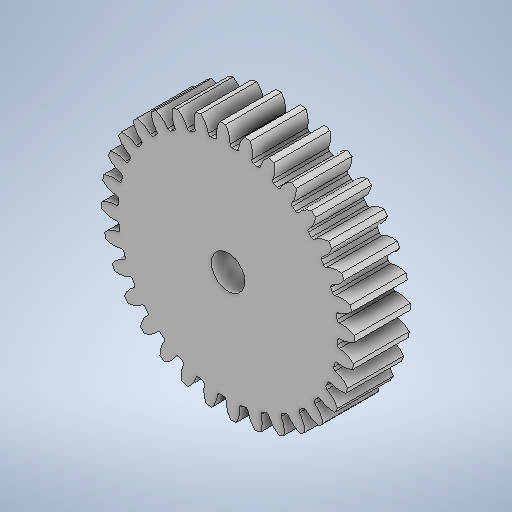
# Autodesk Inventor part: gear32
Saved by Autodesk Inventor 2025.1 (Build 291241000, 241)
## iProperties
Created: 2024-11-04
Part Number: gear32
Material: Generic
Document SubType Name: Modeling
Designer: rishi
Density: 1 g/cm^3
Appearance: Default
Author: rishi
Autodesk Inventor part; units mm, degrees
ref_plane "YZ Plane" through (0, 0, 0) normal (1, 0, 0) x (0, 1, 0)
ref_plane "XZ Plane" through (0, 0, 0) normal (0, 1, 0) x (-1, 0, 0)
ref_plane "XY Plane" through (0, 0, 0) normal (0, 0, 1) x (1, 0, 0)
sketch "Sketch1" plane through (0, 0, 0) normal (0, 0, 1) x (1, 0, 0)
  arc A0 (0.375172, 28.714431) -> (0.375938, 28.717754) centre (-5.995256, 30.18306) ccw
  arc A1 (0.541208, 30.065293) -> (-0.682771, 33.993144) centre (-5.995256, 30.18306) ccw
  arc A2 (0.541208, 30.065293) -> (1.115535, 29.478901) centre (1.111711, 30.049607) ccw
  arc A3 (0.255749, 26.188813) -> (0.375172, 26.259051) centre (-2.99886, 31.859172) ccw
  arc A4 (-2.20376, 33.928505) -> (-3.090042, 29.910974) centre (3.413346, 30.582826) ccw
  arc A5 (-3.587273, 29.281077) -> (-3.090042, 29.910974) centre (-3.656607, 29.84701) ccw
  arc A6 (-3.031796, 29.343794) -> (-3.031451, 29.343829) centre (-3.090042, 29.910974) ccw
  arc A7 (-0.682771, 33.993144) -> (-2.20376, 33.928505) centre (0, 0) ccw
  arc A8 (-0.682771, 33.993144) -> (-2.20376, 33.928505) centre (0, 0) ccw
  arc A9 (-11.19341, 27.293911) -> (-11.334874, 27.235466) centre (0, 0) ccw
  arc A10 (1.115535, 29.478901) -> (-3.587273, 29.281077) centre (0, 0) ccw
  arc A11 (-7.301386, 33.206773) -> (-8.780538, 32.846646) centre (0, 0) ccw
  arc A12 (-5.334639, 29.593181) -> (-7.301386, 33.206773) centre (-11.768482, 28.433485) ccw
  arc A13 (-5.334639, 29.593181) -> (-4.656948, 29.130102) centre (-4.772037, 29.689096) ccw
  arc A14 (-4.656948, 29.130102) -> (-9.2308, 28.018607) centre (0, 0) ccw
  arc A15 (-9.2308, 28.018607) -> (-8.866009, 28.733406) centre (-9.409209, 28.560139) ccw
  arc A16 (-8.780538, 32.846646) -> (-8.866009, 28.733406) centre (-2.618654, 30.661097) ccw
  arc A17 (-13.639412, 31.144284) -> (-15.019885, 30.502509) centre (0, 0) ccw
  arc A18 (-11.005479, 27.98382) -> (-13.639412, 31.144284) centre (-17.089451, 25.591226) ccw
  arc A19 (-11.005479, 27.98382) -> (-10.250467, 27.66185) centre (-10.472399, 28.18765) ccw
  arc A20 (-10.250467, 27.66185) -> (-14.519591, 25.679398) centre (0, 0) ccw
  arc A21 (-14.519591, 25.679398) -> (-14.301261, 26.451629) centre (-14.80022, 26.175719) ccw
  arc A22 (-15.019885, 30.502509) -> (-14.301261, 26.451629) centre (-8.55002, 29.561078) ccw
  arc A23 (-19.453283, 27.884939) -> (-20.682027, 26.986177) centre (0, 0) ccw
  arc A24 (-16.253384, 25.299057) -> (-19.453283, 27.884939) centre (-21.753683, 21.765511) ccw
  arc A25 (-16.253384, 25.299057) -> (-15.450066, 25.130568) centre (-15.770313, 25.602968) ccw
  arc A26 (-15.450066, 25.130568) -> (-19.250403, 22.353344) centre (0, 0) ccw
  arc A27 (-19.250403, 22.353344) -> (-19.186923, 23.153331) centre (-19.622467, 22.78538) ccw
  arc A28 (-20.682027, 26.986177) -> (-19.186923, 23.153331) centre (-14.152814, 27.325044) ccw
  arc A29 (-24.519575, 23.55399) -> (-25.549369, 22.432782) centre (0, 0) ccw
  arc A30 (-20.876681, 21.642065) -> (-24.519575, 23.55399) centre (-25.581932, 17.10336) ccw
  arc A31 (-20.876681, 21.642065) -> (-20.055928, 21.633533) centre (-20.462182, 22.034379) ccw
  arc A32 (-20.055928, 21.633533) -> (-23.241433, 18.168263) centre (0, 0) ccw
  arc A33 (-23.241433, 18.168263) -> (-23.335243, 18.965263) centre (-23.690634, 18.519412) ccw
  arc A34 (-25.549369, 22.432782) -> (-23.335243, 18.965263) centre (-19.211724, 24.038924) ccw
  arc A35 (-28.643594, 18.317875) -> (-29.434864, 17.017308) centre (0, 0) ccw
  arc A36 (-24.697699, 17.15338) -> (-28.643594, 18.317875) centre (-28.427083, 11.783937) ccw
  arc A37 (-24.697699, 17.15338) -> (-23.891052, 17.305133) centre (-24.367701, 17.619021) ccw
  arc A38 (-23.891052, 17.305133) -> (-26.339308, 13.284986) centre (0, 0) ccw
  arc A39 (-26.339308, 13.284986) -> (-26.586802, 14.048371) centre (-26.848383, 13.541753) ccw
  arc A40 (-29.434864, 17.017308) -> (-26.586802, 14.048371) centre (-23.532337, 19.829002) ccw
  arc A41 (-31.666855, 12.377814) -> (-32.189194, 10.947868) centre (0, 0) ccw
  arc A42 (-27.569598, 12.005501) -> (-31.666855, 12.377814) centre (-30.179796, 6.011663) ccw
  arc A43 (-27.569598, 12.005501) -> (-26.808056, 12.311707) centre (-27.336783, 12.526574) ccw
  arc A44 (-26.808056, 12.311707) -> (-28.424978, 7.891175) centre (0, 0) ccw
  arc A45 (-28.424978, 7.891175) -> (-28.816645, 8.591608) centre (-28.974364, 8.043692) ccw
  arc A46 (-32.189194, 10.947868) -> (-28.816645, 8.591608) centre (-26.948616, 14.857062) ccw
  arc A47 (-33.473177, 5.962081) -> (-33.70651, 4.457708) centre (0, 0) ccw
  arc A48 (-29.382012, 6.396257) -> (-33.473177, 5.962081) centre (-30.772717, 0.008364) ccw
  arc A49 (-29.382012, 6.396257) -> (-28.694842, 6.845149) centre (-29.255328, 6.952737) ccw
  arc A50 (-28.694842, 6.845149) -> (-29.418292, 2.19411) centre (0, 0) ccw
  arc A51 (-29.418292, 2.19411) -> (-29.939081, 2.804674) centre (-29.986876, 2.236517) ccw
  arc A52 (-33.70651, 4.457708) -> (-29.939081, 2.804674) centre (-29.329275, 9.314173) ccw
  arc A53 (-33.993144, -0.682771) -> (-33.928505, -2.20376) centre (0, 0) ccw
  arc A54 (-30.065293, 0.541208) -> (-33.993144, -0.682771) centre (-30.18306, -5.995256) ccw
  arc A55 (-30.065293, 0.541208) -> (-29.478901, 1.115535) centre (-30.049607, 1.111711) ccw
  arc A56 (-29.478901, 1.115535) -> (-29.281077, -3.587273) centre (0, 0) ccw
  arc A57 (-29.281077, -3.587273) -> (-29.910974, -3.090042) centre (-29.84701, -3.656607) ccw
  arc A58 (-33.928505, -2.20376) -> (-29.910974, -3.090042) centre (-30.582826, 3.413346) ccw
  arc A59 (-33.206773, -7.301386) -> (-32.846646, -8.780538) centre (0, 0) ccw
  arc A60 (-29.593181, -5.334639) -> (-33.206773, -7.301386) centre (-28.433485, -11.768482) ccw
  arc A61 (-29.593181, -5.334639) -> (-29.130102, -4.656948) centre (-29.689096, -4.772037) ccw
  arc A62 (-29.130102, -4.656948) -> (-28.018607, -9.2308) centre (0, 0) ccw
  arc A63 (-28.018607, -9.2308) -> (-28.733406, -8.866009) centre (-28.560139, -9.409209) ccw
  arc A64 (-32.846646, -8.780538) -> (-28.733406, -8.866009) centre (-30.661097, -2.618654) ccw
  arc A65 (-31.144284, -13.639412) -> (-30.502509, -15.019885) centre (0, 0) ccw
  arc A66 (-27.98382, -11.005479) -> (-31.144284, -13.639412) centre (-25.591226, -17.089451) ccw
  arc A67 (-27.98382, -11.005479) -> (-27.66185, -10.250467) centre (-28.18765, -10.472399) ccw
  arc A68 (-27.66185, -10.250467) -> (-25.679398, -14.519591) centre (0, 0) ccw
  arc A69 (-25.679398, -14.519591) -> (-26.451629, -14.301261) centre (-26.175719, -14.80022) ccw
  arc A70 (-30.502509, -15.019885) -> (-26.451629, -14.301261) centre (-29.561078, -8.55002) ccw
  arc A71 (-27.884939, -19.453283) -> (-26.986177, -20.682027) centre (0, 0) ccw
  arc A72 (-25.299057, -16.253384) -> (-27.884939, -19.453283) centre (-21.765511, -21.753683) ccw
  arc A73 (-25.299057, -16.253384) -> (-25.130568, -15.450066) centre (-25.602968, -15.770313) ccw
  arc A74 (-25.130568, -15.450066) -> (-22.353344, -19.250403) centre (0, 0) ccw
  arc A75 (-22.353344, -19.250403) -> (-23.153331, -19.186923) centre (-22.78538, -19.622467) ccw
  arc A76 (-26.986177, -20.682027) -> (-23.153331, -19.186923) centre (-27.325044, -14.152814) ccw
  arc A77 (-23.55399, -24.519575) -> (-22.432782, -25.549369) centre (0, 0) ccw
  arc A78 (-21.642065, -20.876681) -> (-23.55399, -24.519575) centre (-17.10336, -25.581932) ccw
  arc A79 (-21.642065, -20.876681) -> (-21.633533, -20.055928) centre (-22.034379, -20.462182) ccw
  arc A80 (-21.633533, -20.055928) -> (-18.168263, -23.241433) centre (0, 0) ccw
  arc A81 (-18.168263, -23.241433) -> (-18.965263, -23.335243) centre (-18.519412, -23.690634) ccw
  arc A82 (-22.432782, -25.549369) -> (-18.965263, -23.335243) centre (-24.038924, -19.211724) ccw
  arc A83 (-18.317875, -28.643594) -> (-17.017308, -29.434864) centre (0, 0) ccw
  arc A84 (-17.15338, -24.697699) -> (-18.317875, -28.643594) centre (-11.783937, -28.427083) ccw
  arc A85 (-17.15338, -24.697699) -> (-17.305133, -23.891052) centre (-17.619021, -24.367701) ccw
  arc A86 (-17.305133, -23.891052) -> (-13.284986, -26.339308) centre (0, 0) ccw
  arc A87 (-13.284986, -26.339308) -> (-14.048371, -26.586802) centre (-13.541753, -26.848383) ccw
  arc A88 (-17.017308, -29.434864) -> (-14.048371, -26.586802) centre (-19.829002, -23.532337) ccw
  arc A89 (-12.377814, -31.666855) -> (-10.947868, -32.189194) centre (0, 0) ccw
  arc A90 (-12.005501, -27.569598) -> (-12.377814, -31.666855) centre (-6.011663, -30.179796) ccw
  arc A91 (-12.005501, -27.569598) -> (-12.311707, -26.808056) centre (-12.526574, -27.336783) ccw
  arc A92 (-12.311707, -26.808056) -> (-7.891175, -28.424978) centre (0, 0) ccw
  arc A93 (-7.891175, -28.424978) -> (-8.591608, -28.816645) centre (-8.043692, -28.974364) ccw
  arc A94 (-10.947868, -32.189194) -> (-8.591608, -28.816645) centre (-14.857062, -26.948616) ccw
  arc A95 (-5.962081, -33.473177) -> (-4.457708, -33.70651) centre (0, 0) ccw
  arc A96 (-6.396257, -29.382012) -> (-5.962081, -33.473177) centre (-0.008364, -30.772717) ccw
  arc A97 (-6.396257, -29.382012) -> (-6.845149, -28.694842) centre (-6.952737, -29.255328) ccw
  arc A98 (-6.845149, -28.694842) -> (-2.19411, -29.418292) centre (0, 0) ccw
  arc A99 (-2.19411, -29.418292) -> (-2.804674, -29.939081) centre (-2.236517, -29.986876) ccw
  arc A100 (-4.457708, -33.70651) -> (-2.804674, -29.939081) centre (-9.314173, -29.329275) ccw
  arc A101 (0.682771, -33.993144) -> (2.20376, -33.928505) centre (0, 0) ccw
  arc A102 (-0.541208, -30.065293) -> (0.682771, -33.993144) centre (5.995256, -30.18306) ccw
  arc A103 (-0.541208, -30.065293) -> (-1.115535, -29.478901) centre (-1.111711, -30.049607) ccw
  arc A104 (-1.115535, -29.478901) -> (3.587273, -29.281077) centre (0, 0) ccw
  arc A105 (3.587273, -29.281077) -> (3.090042, -29.910974) centre (3.656607, -29.84701) ccw
  arc A106 (2.20376, -33.928505) -> (3.090042, -29.910974) centre (-3.413346, -30.582826) ccw
  arc A107 (7.301386, -33.206773) -> (8.780538, -32.846646) centre (0, 0) ccw
  arc A108 (5.334639, -29.593181) -> (7.301386, -33.206773) centre (11.768482, -28.433485) ccw
  arc A109 (5.334639, -29.593181) -> (4.656948, -29.130102) centre (4.772037, -29.689096) ccw
  arc A110 (4.656948, -29.130102) -> (9.2308, -28.018607) centre (0, 0) ccw
  arc A111 (9.2308, -28.018607) -> (8.866009, -28.733406) centre (9.409209, -28.560139) ccw
  arc A112 (8.780538, -32.846646) -> (8.866009, -28.733406) centre (2.618654, -30.661097) ccw
  arc A113 (13.639412, -31.144284) -> (15.019885, -30.502509) centre (0, 0) ccw
  arc A114 (11.005479, -27.98382) -> (13.639412, -31.144284) centre (17.089451, -25.591226) ccw
  arc A115 (11.005479, -27.98382) -> (10.250467, -27.66185) centre (10.472399, -28.18765) ccw
  arc A116 (10.250467, -27.66185) -> (14.519591, -25.679398) centre (0, 0) ccw
  arc A117 (14.519591, -25.679398) -> (14.301261, -26.451629) centre (14.80022, -26.175719) ccw
  arc A118 (15.019885, -30.502509) -> (14.301261, -26.451629) centre (8.55002, -29.561078) ccw
  arc A119 (19.453283, -27.884939) -> (20.682027, -26.986177) centre (0, 0) ccw
  arc A120 (16.253384, -25.299057) -> (19.453283, -27.884939) centre (21.753683, -21.765511) ccw
  arc A121 (16.253384, -25.299057) -> (15.450066, -25.130568) centre (15.770313, -25.602968) ccw
  arc A122 (15.450066, -25.130568) -> (19.250403, -22.353344) centre (0, 0) ccw
  arc A123 (19.250403, -22.353344) -> (19.186923, -23.153331) centre (19.622467, -22.78538) ccw
  arc A124 (20.682027, -26.986177) -> (19.186923, -23.153331) centre (14.152814, -27.325044) ccw
  arc A125 (24.519575, -23.55399) -> (25.549369, -22.432782) centre (0, 0) ccw
  arc A126 (20.876681, -21.642065) -> (24.519575, -23.55399) centre (25.581932, -17.10336) ccw
  arc A127 (20.876681, -21.642065) -> (20.055928, -21.633533) centre (20.462182, -22.034379) ccw
  arc A128 (20.055928, -21.633533) -> (23.241433, -18.168263) centre (0, 0) ccw
  arc A129 (23.241433, -18.168263) -> (23.335243, -18.965263) centre (23.690634, -18.519412) ccw
  arc A130 (25.549369, -22.432782) -> (23.335243, -18.965263) centre (19.211724, -24.038924) ccw
  arc A131 (28.643594, -18.317875) -> (29.434864, -17.017308) centre (0, 0) ccw
  arc A132 (24.697699, -17.15338) -> (28.643594, -18.317875) centre (28.427083, -11.783937) ccw
  arc A133 (24.697699, -17.15338) -> (23.891052, -17.305133) centre (24.367701, -17.619021) ccw
  arc A134 (23.891052, -17.305133) -> (26.339308, -13.284986) centre (0, 0) ccw
  arc A135 (26.339308, -13.284986) -> (26.586802, -14.048371) centre (26.848383, -13.541753) ccw
  arc A136 (29.434864, -17.017308) -> (26.586802, -14.048371) centre (23.532337, -19.829002) ccw
  arc A137 (31.666855, -12.377814) -> (32.189194, -10.947868) centre (0, 0) ccw
  arc A138 (27.569598, -12.005501) -> (31.666855, -12.377814) centre (30.179796, -6.011663) ccw
  arc A139 (27.569598, -12.005501) -> (26.808056, -12.311707) centre (27.336783, -12.526574) ccw
  arc A140 (26.808056, -12.311707) -> (28.424978, -7.891175) centre (0, 0) ccw
  arc A141 (28.424978, -7.891175) -> (28.816645, -8.591608) centre (28.974364, -8.043692) ccw
  arc A142 (32.189194, -10.947868) -> (28.816645, -8.591608) centre (26.948616, -14.857062) ccw
  arc A143 (33.473177, -5.962081) -> (33.70651, -4.457708) centre (0, 0) ccw
  arc A144 (29.382012, -6.396257) -> (33.473177, -5.962081) centre (30.772717, -0.008364) ccw
  arc A145 (29.382012, -6.396257) -> (28.694842, -6.845149) centre (29.255328, -6.952737) ccw
  arc A146 (28.694842, -6.845149) -> (29.418292, -2.19411) centre (0, 0) ccw
  arc A147 (29.418292, -2.19411) -> (29.939081, -2.804674) centre (29.986876, -2.236517) ccw
  arc A148 (33.70651, -4.457708) -> (29.939081, -2.804674) centre (29.329275, -9.314173) ccw
  arc A149 (33.993144, 0.682771) -> (33.928505, 2.20376) centre (0, 0) ccw
  arc A150 (30.065293, -0.541208) -> (33.993144, 0.682771) centre (30.18306, 5.995256) ccw
  arc A151 (30.065293, -0.541208) -> (29.478901, -1.115535) centre (30.049607, -1.111711) ccw
  arc A152 (29.478901, -1.115535) -> (29.281077, 3.587273) centre (0, 0) ccw
  arc A153 (29.281077, 3.587273) -> (29.910974, 3.090042) centre (29.84701, 3.656607) ccw
  arc A154 (33.928505, 2.20376) -> (29.910974, 3.090042) centre (30.582826, -3.413346) ccw
  arc A155 (33.206773, 7.301386) -> (32.846646, 8.780538) centre (0, 0) ccw
  arc A156 (29.593181, 5.334639) -> (33.206773, 7.301386) centre (28.433485, 11.768482) ccw
  arc A157 (29.593181, 5.334639) -> (29.130102, 4.656948) centre (29.689096, 4.772037) ccw
  arc A158 (29.130102, 4.656948) -> (28.018607, 9.2308) centre (0, 0) ccw
  arc A159 (28.018607, 9.2308) -> (28.733406, 8.866009) centre (28.560139, 9.409209) ccw
  arc A160 (32.846646, 8.780538) -> (28.733406, 8.866009) centre (30.661097, 2.618654) ccw
  arc A161 (31.144284, 13.639412) -> (30.502509, 15.019885) centre (0, 0) ccw
  arc A162 (27.98382, 11.005479) -> (31.144284, 13.639412) centre (25.591226, 17.089451) ccw
  arc A163 (27.98382, 11.005479) -> (27.66185, 10.250467) centre (28.18765, 10.472399) ccw
  arc A164 (27.66185, 10.250467) -> (25.679398, 14.519591) centre (0, 0) ccw
  arc A165 (25.679398, 14.519591) -> (26.451629, 14.301261) centre (26.175719, 14.80022) ccw
  arc A166 (30.502509, 15.019885) -> (26.451629, 14.301261) centre (29.561078, 8.55002) ccw
  arc A167 (27.884939, 19.453283) -> (26.986177, 20.682027) centre (0, 0) ccw
  arc A168 (25.299057, 16.253384) -> (27.884939, 19.453283) centre (21.765511, 21.753683) ccw
  arc A169 (25.299057, 16.253384) -> (25.130568, 15.450066) centre (25.602968, 15.770313) ccw
  arc A170 (25.130568, 15.450066) -> (22.353344, 19.250403) centre (0, 0) ccw
  arc A171 (22.353344, 19.250403) -> (23.153331, 19.186923) centre (22.78538, 19.622467) ccw
  arc A172 (26.986177, 20.682027) -> (23.153331, 19.186923) centre (27.325044, 14.152814) ccw
  arc A173 (23.55399, 24.519575) -> (22.432782, 25.549369) centre (0, 0) ccw
  arc A174 (21.642065, 20.876681) -> (23.55399, 24.519575) centre (17.10336, 25.581932) ccw
  arc A175 (21.642065, 20.876681) -> (21.633533, 20.055928) centre (22.034379, 20.462182) ccw
  arc A176 (21.633533, 20.055928) -> (18.168263, 23.241433) centre (0, 0) ccw
  arc A177 (18.168263, 23.241433) -> (18.965263, 23.335243) centre (18.519412, 23.690634) ccw
  arc A178 (22.432782, 25.549369) -> (18.965263, 23.335243) centre (24.038924, 19.211724) ccw
  arc A179 (18.317875, 28.643594) -> (17.017308, 29.434864) centre (0, 0) ccw
  arc A180 (17.15338, 24.697699) -> (18.317875, 28.643594) centre (11.783937, 28.427083) ccw
  arc A181 (17.15338, 24.697699) -> (17.305133, 23.891052) centre (17.619021, 24.367701) ccw
  arc A182 (17.305133, 23.891052) -> (13.284986, 26.339308) centre (0, 0) ccw
  arc A183 (13.284986, 26.339308) -> (14.048371, 26.586802) centre (13.541753, 26.848383) ccw
  arc A184 (17.017308, 29.434864) -> (14.048371, 26.586802) centre (19.829002, 23.532337) ccw
  arc A185 (12.377814, 31.666855) -> (10.947868, 32.189194) centre (0, 0) ccw
  arc A186 (12.005501, 27.569598) -> (12.377814, 31.666855) centre (6.011663, 30.179796) ccw
  arc A187 (12.005501, 27.569598) -> (12.311707, 26.808056) centre (12.526574, 27.336783) ccw
  arc A188 (12.311707, 26.808056) -> (7.891175, 28.424978) centre (0, 0) ccw
  arc A189 (7.891175, 28.424978) -> (8.591608, 28.816645) centre (8.043692, 28.974364) ccw
  arc A190 (10.947868, 32.189194) -> (8.591608, 28.816645) centre (14.857062, 26.948616) ccw
  arc A191 (5.962081, 33.473177) -> (4.457708, 33.70651) centre (0, 0) ccw
  arc A192 (6.396257, 29.382012) -> (5.962081, 33.473177) centre (0.008364, 30.772717) ccw
  arc A193 (6.396257, 29.382012) -> (6.845149, 28.694842) centre (6.952737, 29.255328) ccw
  arc A194 (6.845149, 28.694842) -> (2.19411, 29.418292) centre (0, 0) ccw
  arc A195 (2.19411, 29.418292) -> (2.804674, 29.939081) centre (2.236517, 29.986876) ccw
  arc A196 (4.457708, 33.70651) -> (2.804674, 29.939081) centre (9.314173, 29.329275) ccw
  circle A197 centre (0, 0) radius 29.5
  arc A198 (3.5, 2.828427) -> (3.5, -2.828427) centre (0, 0) ccw
  line L0 (3.5, -2.828427) -> (3.5, 2.828427)
  point P0 (0, 34)
  point P1 (0, 34)
  point P2 (0, 32.79)
  point P3 (-6.397012, 32.159949)
  point P4 (-8.6979, 28.188589)
  point P5 (-12.54819, 30.29401)
  point P6 (-14.030093, 25.950077)
  point P7 (-18.217148, 27.263889)
  point P8 (-18.823118, 22.714318)
  point P9 (-23.186031, 23.186031)
  point P10 (-22.89278, 18.605661)
  point P11 (-27.263889, 18.217148)
  point P12 (-26.082686, 13.781998)
  point P13 (-30.29401, 12.54819)
  point P14 (-28.270249, 8.428701)
  point P15 (-32.159949, 6.397012)
  point P16 (-29.371402, 2.751494)
  point P17 (-32.79, 0)
  point P18 (-29.343829, -3.031451)
  point P19 (-32.159949, -6.397012)
  point P20 (-28.188589, -8.6979)
  point P21 (-30.29401, -12.54819)
  point P22 (-25.950077, -14.030093)
  point P23 (-27.263889, -18.217148)
  point P24 (-22.714318, -18.823118)
  point P25 (-23.186031, -23.186031)
  point P26 (-18.605661, -22.89278)
  point P27 (-18.217148, -27.263889)
  point P28 (-13.781998, -26.082686)
  point P29 (-12.54819, -30.29401)
  point P30 (-8.428701, -28.270249)
  point P31 (-6.397012, -32.159949)
  point P32 (-2.751494, -29.371402)
  point P33 (0, -32.79)
  point P34 (3.031451, -29.343829)
  point P35 (6.397012, -32.159949)
  point P36 (8.6979, -28.188589)
  point P37 (12.54819, -30.29401)
  point P38 (14.030093, -25.950077)
  point P39 (18.217148, -27.263889)
  point P40 (18.823118, -22.714318)
  point P41 (23.186031, -23.186031)
  point P42 (22.89278, -18.605661)
  point P43 (27.263889, -18.217148)
  point P44 (26.082686, -13.781998)
  point P45 (30.29401, -12.54819)
  point P46 (28.270249, -8.428701)
  point P47 (32.159949, -6.397012)
  point P48 (29.371402, -2.751494)
  point P49 (32.79, 0)
  point P50 (29.343829, 3.031451)
  point P51 (32.159949, 6.397012)
  point P52 (28.188589, 8.6979)
  point P53 (30.29401, 12.54819)
  point P54 (25.950077, 14.030093)
  point P55 (27.263889, 18.217148)
  point P56 (22.714318, 18.823118)
  point P57 (23.186031, 23.186031)
  point P58 (18.605661, 22.89278)
  point P59 (18.217148, 27.263889)
  point P60 (13.781998, 26.082686)
  point P61 (12.54819, 30.29401)
  point P62 (8.428701, 28.270249)
  point P63 (6.397012, 32.159949)
  point P64 (2.751494, 29.371402)
  point P65 (-29.418292, 2.19411)
  point P66 (-29.478901, 1.115535)
  point P67 (-29.480743, 1.065728)
  point P68 (-29.281077, -3.587273)
  point P69 (-29.130102, -4.656948)
  point P70 (-29.122192, -4.706157)
  point P71 (-28.018607, -9.2308)
  point P72 (-27.66185, -10.250467)
  point P73 (-27.644492, -10.297188)
  point P74 (-25.679398, -14.519591)
  point P75 (-25.130568, -15.450066)
  point P76 (-25.104429, -15.492503)
  point P77 (-22.353344, -19.250403)
  point P78 (-21.633533, -20.055928)
  point P79 (-21.599617, -20.09245)
  point P80 (-18.168263, -23.241433)
  point P81 (-17.305133, -23.891052)
  point P82 (-17.264744, -23.920255)
  point P83 (-13.284986, -26.339308)
  point P84 (-12.311707, -26.808056)
  point P85 (-12.266396, -26.828819)
  point P86 (-7.891175, -28.424978)
  point P87 (-6.845149, -28.694842)
  point P88 (-6.796658, -28.706366)
  point P89 (-2.19411, -29.418292)
  point P90 (-1.115535, -29.478901)
  point P91 (-1.065728, -29.480743)
  point P92 (3.587273, -29.281077)
  point P93 (4.656948, -29.130102)
  point P94 (4.706157, -29.122192)
  point P95 (9.2308, -28.018607)
  point P96 (10.250467, -27.66185)
  point P97 (10.297188, -27.644492)
  point P98 (14.519591, -25.679398)
  point P99 (15.450066, -25.130568)
  point P100 (15.492503, -25.104429)
  point P101 (19.250403, -22.353344)
  point P102 (20.055928, -21.633533)
  point P103 (20.09245, -21.599617)
  point P104 (23.241433, -18.168263)
  point P105 (23.891052, -17.305133)
  point P106 (23.920255, -17.264744)
  point P107 (26.339308, -13.284986)
  point P108 (26.808056, -12.311707)
  point P109 (26.828819, -12.266396)
  point P110 (28.424978, -7.891175)
  point P111 (28.694842, -6.845149)
  point P112 (28.706366, -6.796658)
  point P113 (29.418292, -2.19411)
  point P114 (29.478901, -1.115535)
  point P115 (29.480743, -1.065728)
  point P116 (29.281077, 3.587273)
  point P117 (29.130102, 4.656948)
  point P118 (29.122192, 4.706157)
  point P119 (28.018607, 9.2308)
  point P120 (27.66185, 10.250467)
  point P121 (27.644492, 10.297188)
  point P122 (25.679398, 14.519591)
  point P123 (25.130568, 15.450066)
  point P124 (25.104429, 15.492503)
  point P125 (22.353344, 19.250403)
  point P126 (21.633533, 20.055928)
  point P127 (21.599617, 20.09245)
  point P128 (18.168263, 23.241433)
  point P129 (17.305133, 23.891052)
  point P130 (17.264744, 23.920255)
  point P131 (13.284986, 26.339308)
  point P132 (12.311707, 26.808056)
  point P133 (12.266396, 26.828819)
  point P134 (7.891175, 28.424978)
  point P135 (6.845149, 28.694842)
  point P136 (6.796658, 28.706366)
  point P137 (2.19411, 29.418292)
  point P138 (1.115535, 29.478901)
  point P139 (1.065728, 29.480743)
  point P140 (-3.587273, 29.281077)
  point P141 (-4.656948, 29.130102)
  point P142 (-4.706157, 29.122192)
  point P143 (-9.2308, 28.018607)
  point P144 (-10.250467, 27.66185)
  point P145 (-10.297188, 27.644492)
  point P146 (-14.519591, 25.679398)
  point P147 (-15.450066, 25.130568)
  point P148 (-15.492503, 25.104429)
  point P149 (-19.250403, 22.353344)
  point P150 (-20.055928, 21.633533)
  point P151 (-20.09245, 21.599617)
  point P152 (-23.241433, 18.168263)
  point P153 (-23.891052, 17.305133)
  point P154 (-23.920255, 17.264744)
  point P155 (-26.339308, 13.284986)
  point P156 (-26.808056, 12.311707)
  point P157 (-26.828819, 12.266396)
  point P158 (-28.424978, 7.891175)
  point P159 (-28.694842, 6.845149)
  point P160 (-28.706366, 6.796658)
  dimension "d12" = 360
  constraints: 460 point on circle, 198 centre point, 6 coincident, 2 end point, 1 vertical, 644 other
sketch "Sketch1 outline for Extrusion1" plane through (0, 0, 0) normal (0, 0, 1) x (1, 0, 0)
  arc A0 (-29.418292, 2.19411) -> (-29.478901, 1.115535) centre (0, 0) ccw
  arc A1 (-29.939081, 2.804674) -> (-29.418292, 2.19411) centre (-29.986876, 2.236517) cw
  arc A2 (-33.70651, 4.457708) -> (-29.939081, 2.804674) centre (-29.329275, 9.314173) ccw
  arc A3 (-33.473177, 5.962081) -> (-33.70651, 4.457708) centre (0, 0) ccw
  arc A4 (-29.382012, 6.396257) -> (-33.473177, 5.962081) centre (-30.772717, 0.008364) ccw
  arc A5 (-28.706366, 6.796658) -> (-29.382012, 6.396257) centre (-29.255328, 6.952737) cw
  arc A6 (-28.694842, 6.845149) -> (-28.706366, 6.796658) centre (-0.000002, 0.000001) ccw
  arc A7 (-28.424978, 7.891175) -> (-28.694842, 6.845149) centre (0, 0) ccw
  arc A8 (-28.816645, 8.591608) -> (-28.424978, 7.891175) centre (-28.974364, 8.043692) cw
  arc A9 (-32.189194, 10.947868) -> (-28.816645, 8.591608) centre (-26.948616, 14.857062) ccw
  arc A10 (-31.666855, 12.377814) -> (-32.189194, 10.947868) centre (0, 0) ccw
  arc A11 (-27.569598, 12.005501) -> (-31.666855, 12.377814) centre (-30.179796, 6.011663) ccw
  arc A12 (-26.828819, 12.266396) -> (-27.569598, 12.005501) centre (-27.336783, 12.526574) cw
  arc A13 (-26.808056, 12.311707) -> (-26.828819, 12.266396) centre (-0.000002, 0.000001) ccw
  arc A14 (-26.339308, 13.284986) -> (-26.808056, 12.311707) centre (0, 0) ccw
  arc A15 (-26.586802, 14.048371) -> (-26.339308, 13.284986) centre (-26.848383, 13.541753) cw
  arc A16 (-29.434864, 17.017308) -> (-26.586802, 14.048371) centre (-23.532337, 19.829002) ccw
  arc A17 (-28.643594, 18.317875) -> (-29.434864, 17.017308) centre (0, 0) ccw
  arc A18 (-24.697699, 17.15338) -> (-28.643594, 18.317875) centre (-28.427083, 11.783937) ccw
  arc A19 (-23.920255, 17.264744) -> (-24.697699, 17.15338) centre (-24.367701, 17.619021) cw
  arc A20 (-23.891052, 17.305133) -> (-23.920255, 17.264744) centre (-0.000002, 0.000001) ccw
  arc A21 (-23.241433, 18.168263) -> (-23.891052, 17.305133) centre (0, 0) ccw
  arc A22 (-23.335243, 18.965263) -> (-23.241433, 18.168263) centre (-23.690634, 18.519412) cw
  arc A23 (-25.549369, 22.432782) -> (-23.335243, 18.965263) centre (-19.211724, 24.038924) ccw
  arc A24 (-24.519575, 23.55399) -> (-25.549369, 22.432782) centre (0, 0) ccw
  arc A25 (-20.876681, 21.642065) -> (-24.519575, 23.55399) centre (-25.581932, 17.10336) ccw
  arc A26 (-20.09245, 21.599617) -> (-20.876681, 21.642065) centre (-20.462182, 22.034379) cw
  arc A27 (-20.055928, 21.633533) -> (-20.09245, 21.599617) centre (-0.000002, 0.000002) ccw
  arc A28 (-19.250403, 22.353344) -> (-20.055928, 21.633533) centre (0, 0) ccw
  arc A29 (-19.186923, 23.153331) -> (-19.250403, 22.353344) centre (-19.622467, 22.78538) cw
  arc A30 (-20.682027, 26.986177) -> (-19.186923, 23.153331) centre (-14.152814, 27.325044) ccw
  arc A31 (-19.453283, 27.884939) -> (-20.682027, 26.986177) centre (0, 0) ccw
  arc A32 (-16.253384, 25.299057) -> (-19.453283, 27.884939) centre (-21.753683, 21.765511) ccw
  arc A33 (-15.492503, 25.104429) -> (-16.253384, 25.299057) centre (-15.770313, 25.602968) cw
  arc A34 (-15.450066, 25.130568) -> (-15.492503, 25.104429) centre (-0.000001, 0.000002) ccw
  arc A35 (-14.519591, 25.679398) -> (-15.450066, 25.130568) centre (0, 0) ccw
  arc A36 (-14.301261, 26.451629) -> (-14.519591, 25.679398) centre (-14.80022, 26.175719) cw
  arc A37 (-15.019885, 30.502509) -> (-14.301261, 26.451629) centre (-8.55002, 29.561078) ccw
  arc A38 (-13.639412, 31.144284) -> (-15.019885, 30.502509) centre (0, 0) ccw
  arc A39 (-11.005479, 27.98382) -> (-13.639412, 31.144284) centre (-17.089451, 25.591226) ccw
  arc A40 (-10.297188, 27.644492) -> (-11.005479, 27.98382) centre (-10.472399, 28.18765) cw
  arc A41 (-10.250467, 27.66185) -> (-10.297188, 27.644492) centre (-0.000001, 0.000002) ccw
  arc A42 (-9.2308, 28.018607) -> (-10.250467, 27.66185) centre (0, 0) ccw
  arc A43 (-8.866009, 28.733406) -> (-9.2308, 28.018607) centre (-9.409209, 28.560139) cw
  arc A44 (-8.780538, 32.846646) -> (-8.866009, 28.733406) centre (-2.618654, 30.661097) ccw
  arc A45 (-7.301386, 33.206773) -> (-8.780538, 32.846646) centre (0, 0) ccw
  arc A46 (-5.334639, 29.593181) -> (-7.301386, 33.206773) centre (-11.768482, 28.433485) ccw
  arc A47 (-4.706157, 29.122192) -> (-5.334639, 29.593181) centre (-4.772037, 29.689096) cw
  arc A48 (-4.656948, 29.130102) -> (-4.706157, 29.122192) centre (0, 0.000002) ccw
  arc A49 (-3.587273, 29.281077) -> (-4.656948, 29.130102) centre (0, 0) ccw
  arc A50 (-3.090042, 29.910974) -> (-3.587273, 29.281077) centre (-3.656607, 29.84701) cw
  arc A51 (-2.20376, 33.928505) -> (-3.090042, 29.910974) centre (3.413346, 30.582826) ccw
  arc A52 (-0.682771, 33.993144) -> (-2.20376, 33.928505) centre (0, 0) ccw
  arc A53 (0.541208, 30.065293) -> (-0.682771, 33.993144) centre (-5.995256, 30.18306) ccw
  arc A54 (1.065728, 29.480743) -> (0.541208, 30.065293) centre (1.111711, 30.049607) cw
  arc A55 (1.115535, 29.478901) -> (1.065728, 29.480743) centre (0, 0.000002) ccw
  arc A56 (2.19411, 29.418292) -> (1.115535, 29.478901) centre (0, 0) ccw
  arc A57 (2.804674, 29.939081) -> (2.19411, 29.418292) centre (2.236517, 29.986876) cw
  arc A58 (4.457708, 33.70651) -> (2.804674, 29.939081) centre (9.314173, 29.329275) ccw
  arc A59 (5.962081, 33.473177) -> (4.457708, 33.70651) centre (0, 0) ccw
  arc A60 (6.396257, 29.382012) -> (5.962081, 33.473177) centre (0.008364, 30.772717) ccw
  arc A61 (6.796658, 28.706366) -> (6.396257, 29.382012) centre (6.952737, 29.255328) cw
  arc A62 (6.845149, 28.694842) -> (6.796658, 28.706366) centre (0.000001, 0.000002) ccw
  arc A63 (7.891175, 28.424978) -> (6.845149, 28.694842) centre (0, 0) ccw
  arc A64 (8.591608, 28.816645) -> (7.891175, 28.424978) centre (8.043692, 28.974364) cw
  arc A65 (10.947868, 32.189194) -> (8.591608, 28.816645) centre (14.857062, 26.948616) ccw
  arc A66 (12.377814, 31.666855) -> (10.947868, 32.189194) centre (0, 0) ccw
  arc A67 (12.005501, 27.569598) -> (12.377814, 31.666855) centre (6.011663, 30.179796) ccw
  arc A68 (12.266396, 26.828819) -> (12.005501, 27.569598) centre (12.526574, 27.336783) cw
  arc A69 (12.311707, 26.808056) -> (12.266396, 26.828819) centre (0.000001, 0.000002) ccw
  arc A70 (13.284986, 26.339308) -> (12.311707, 26.808056) centre (0, 0) ccw
  arc A71 (14.048371, 26.586802) -> (13.284986, 26.339308) centre (13.541753, 26.848383) cw
  arc A72 (17.017308, 29.434864) -> (14.048371, 26.586802) centre (19.829002, 23.532337) ccw
  arc A73 (18.317875, 28.643594) -> (17.017308, 29.434864) centre (0, 0) ccw
  arc A74 (17.15338, 24.697699) -> (18.317875, 28.643594) centre (11.783937, 28.427083) ccw
  arc A75 (17.264744, 23.920255) -> (17.15338, 24.697699) centre (17.619021, 24.367701) cw
  arc A76 (17.305133, 23.891052) -> (17.264744, 23.920255) centre (0.000001, 0.000002) ccw
  arc A77 (18.168263, 23.241433) -> (17.305133, 23.891052) centre (0, 0) ccw
  arc A78 (18.965263, 23.335243) -> (18.168263, 23.241433) centre (18.519412, 23.690634) cw
  arc A79 (22.432782, 25.549369) -> (18.965263, 23.335243) centre (24.038924, 19.211724) ccw
  arc A80 (23.55399, 24.519575) -> (22.432782, 25.549369) centre (0, 0) ccw
  arc A81 (21.642065, 20.876681) -> (23.55399, 24.519575) centre (17.10336, 25.581932) ccw
  arc A82 (21.599617, 20.09245) -> (21.642065, 20.876681) centre (22.034379, 20.462182) cw
  arc A83 (21.633533, 20.055928) -> (21.599617, 20.09245) centre (0.000002, 0.000002) ccw
  arc A84 (22.353344, 19.250403) -> (21.633533, 20.055928) centre (0, 0) ccw
  arc A85 (23.153331, 19.186923) -> (22.353344, 19.250403) centre (22.78538, 19.622467) cw
  arc A86 (26.986177, 20.682027) -> (23.153331, 19.186923) centre (27.325044, 14.152814) ccw
  arc A87 (27.884939, 19.453283) -> (26.986177, 20.682027) centre (0, 0) ccw
  arc A88 (25.299057, 16.253384) -> (27.884939, 19.453283) centre (21.765511, 21.753683) ccw
  arc A89 (25.104429, 15.492503) -> (25.299057, 16.253384) centre (25.602968, 15.770313) cw
  arc A90 (25.130568, 15.450066) -> (25.104429, 15.492503) centre (0.000002, 0.000001) ccw
  arc A91 (25.679398, 14.519591) -> (25.130568, 15.450066) centre (0, 0) ccw
  arc A92 (26.451629, 14.301261) -> (25.679398, 14.519591) centre (26.175719, 14.80022) cw
  arc A93 (30.502509, 15.019885) -> (26.451629, 14.301261) centre (29.561078, 8.55002) ccw
  arc A94 (31.144284, 13.639412) -> (30.502509, 15.019885) centre (0, 0) ccw
  arc A95 (27.98382, 11.005479) -> (31.144284, 13.639412) centre (25.591226, 17.089451) ccw
  arc A96 (27.644492, 10.297188) -> (27.98382, 11.005479) centre (28.18765, 10.472399) cw
  arc A97 (27.66185, 10.250467) -> (27.644492, 10.297188) centre (0.000002, 0.000001) ccw
  arc A98 (28.018607, 9.2308) -> (27.66185, 10.250467) centre (0, 0) ccw
  arc A99 (28.733406, 8.866009) -> (28.018607, 9.2308) centre (28.560139, 9.409209) cw
  arc A100 (32.846646, 8.780538) -> (28.733406, 8.866009) centre (30.661097, 2.618654) ccw
  arc A101 (33.206773, 7.301386) -> (32.846646, 8.780538) centre (0, 0) ccw
  arc A102 (29.593181, 5.334639) -> (33.206773, 7.301386) centre (28.433485, 11.768482) ccw
  arc A103 (29.122192, 4.706157) -> (29.593181, 5.334639) centre (29.689096, 4.772037) cw
  arc A104 (29.130102, 4.656948) -> (29.122192, 4.706157) centre (0.000002, 0) ccw
  arc A105 (29.281077, 3.587273) -> (29.130102, 4.656948) centre (0, 0) ccw
  arc A106 (29.910974, 3.090042) -> (29.281077, 3.587273) centre (29.84701, 3.656607) cw
  arc A107 (33.928505, 2.20376) -> (29.910974, 3.090042) centre (30.582826, -3.413346) ccw
  arc A108 (33.993144, 0.682771) -> (33.928505, 2.20376) centre (0, 0) ccw
  arc A109 (30.065293, -0.541208) -> (33.993144, 0.682771) centre (30.18306, 5.995256) ccw
  arc A110 (29.480743, -1.065728) -> (30.065293, -0.541208) centre (30.049607, -1.111711) cw
  arc A111 (29.478901, -1.115535) -> (29.480743, -1.065728) centre (0.000002, 0) ccw
  arc A112 (29.418292, -2.19411) -> (29.478901, -1.115535) centre (0, 0) ccw
  arc A113 (29.939081, -2.804674) -> (29.418292, -2.19411) centre (29.986876, -2.236517) cw
  arc A114 (33.70651, -4.457708) -> (29.939081, -2.804674) centre (29.329275, -9.314173) ccw
  arc A115 (33.473177, -5.962081) -> (33.70651, -4.457708) centre (0, 0) ccw
  arc A116 (29.382012, -6.396257) -> (33.473177, -5.962081) centre (30.772717, -0.008364) ccw
  arc A117 (28.706366, -6.796658) -> (29.382012, -6.396257) centre (29.255328, -6.952737) cw
  arc A118 (28.694842, -6.845149) -> (28.706366, -6.796658) centre (0.000002, -0.000001) ccw
  arc A119 (28.424978, -7.891175) -> (28.694842, -6.845149) centre (0, 0) ccw
  arc A120 (28.816645, -8.591608) -> (28.424978, -7.891175) centre (28.974364, -8.043692) cw
  arc A121 (32.189194, -10.947868) -> (28.816645, -8.591608) centre (26.948616, -14.857062) ccw
  arc A122 (31.666855, -12.377814) -> (32.189194, -10.947868) centre (0, 0) ccw
  arc A123 (27.569598, -12.005501) -> (31.666855, -12.377814) centre (30.179796, -6.011663) ccw
  arc A124 (26.828819, -12.266396) -> (27.569598, -12.005501) centre (27.336783, -12.526574) cw
  arc A125 (26.808056, -12.311707) -> (26.828819, -12.266396) centre (0.000002, -0.000001) ccw
  arc A126 (26.339308, -13.284986) -> (26.808056, -12.311707) centre (0, 0) ccw
  arc A127 (26.586802, -14.048371) -> (26.339308, -13.284986) centre (26.848383, -13.541753) cw
  arc A128 (29.434864, -17.017308) -> (26.586802, -14.048371) centre (23.532337, -19.829002) ccw
  arc A129 (28.643594, -18.317875) -> (29.434864, -17.017308) centre (0, 0) ccw
  arc A130 (24.697699, -17.15338) -> (28.643594, -18.317875) centre (28.427083, -11.783937) ccw
  arc A131 (23.920255, -17.264744) -> (24.697699, -17.15338) centre (24.367701, -17.619021) cw
  arc A132 (23.891052, -17.305133) -> (23.920255, -17.264744) centre (0.000002, -0.000001) ccw
  arc A133 (23.241433, -18.168263) -> (23.891052, -17.305133) centre (0, 0) ccw
  arc A134 (23.335243, -18.965263) -> (23.241433, -18.168263) centre (23.690634, -18.519412) cw
  arc A135 (25.549369, -22.432782) -> (23.335243, -18.965263) centre (19.211724, -24.038924) ccw
  arc A136 (24.519575, -23.55399) -> (25.549369, -22.432782) centre (0, 0) ccw
  arc A137 (20.876681, -21.642065) -> (24.519575, -23.55399) centre (25.581932, -17.10336) ccw
  arc A138 (20.09245, -21.599617) -> (20.876681, -21.642065) centre (20.462182, -22.034379) cw
  arc A139 (20.055928, -21.633533) -> (20.09245, -21.599617) centre (0.000002, -0.000002) ccw
  arc A140 (19.250403, -22.353344) -> (20.055928, -21.633533) centre (0, 0) ccw
  arc A141 (19.186923, -23.153331) -> (19.250403, -22.353344) centre (19.622467, -22.78538) cw
  arc A142 (20.682027, -26.986177) -> (19.186923, -23.153331) centre (14.152814, -27.325044) ccw
  arc A143 (19.453283, -27.884939) -> (20.682027, -26.986177) centre (0, 0) ccw
  arc A144 (16.253384, -25.299057) -> (19.453283, -27.884939) centre (21.753683, -21.765511) ccw
  arc A145 (15.492503, -25.104429) -> (16.253384, -25.299057) centre (15.770313, -25.602968) cw
  arc A146 (15.450066, -25.130568) -> (15.492503, -25.104429) centre (0.000001, -0.000002) ccw
  arc A147 (14.519591, -25.679398) -> (15.450066, -25.130568) centre (0, 0) ccw
  arc A148 (14.301261, -26.451629) -> (14.519591, -25.679398) centre (14.80022, -26.175719) cw
  arc A149 (15.019885, -30.502509) -> (14.301261, -26.451629) centre (8.55002, -29.561078) ccw
  arc A150 (13.639412, -31.144284) -> (15.019885, -30.502509) centre (0, 0) ccw
  arc A151 (11.005479, -27.98382) -> (13.639412, -31.144284) centre (17.089451, -25.591226) ccw
  arc A152 (10.297188, -27.644492) -> (11.005479, -27.98382) centre (10.472399, -28.18765) cw
  arc A153 (10.250467, -27.66185) -> (10.297188, -27.644492) centre (0.000001, -0.000002) ccw
  arc A154 (9.2308, -28.018607) -> (10.250467, -27.66185) centre (0, 0) ccw
  arc A155 (8.866009, -28.733406) -> (9.2308, -28.018607) centre (9.409209, -28.560139) cw
  arc A156 (8.780538, -32.846646) -> (8.866009, -28.733406) centre (2.618654, -30.661097) ccw
  arc A157 (7.301386, -33.206773) -> (8.780538, -32.846646) centre (0, 0) ccw
  arc A158 (5.334639, -29.593181) -> (7.301386, -33.206773) centre (11.768482, -28.433485) ccw
  arc A159 (4.706157, -29.122192) -> (5.334639, -29.593181) centre (4.772037, -29.689096) cw
  arc A160 (4.656948, -29.130102) -> (4.706157, -29.122192) centre (0, -0.000002) ccw
  arc A161 (3.587273, -29.281077) -> (4.656948, -29.130102) centre (0, 0) ccw
  arc A162 (3.090042, -29.910974) -> (3.587273, -29.281077) centre (3.656607, -29.84701) cw
  arc A163 (2.20376, -33.928505) -> (3.090042, -29.910974) centre (-3.413346, -30.582826) ccw
  arc A164 (0.682771, -33.993144) -> (2.20376, -33.928505) centre (0, 0) ccw
  arc A165 (-0.541208, -30.065293) -> (0.682771, -33.993144) centre (5.995256, -30.18306) ccw
  arc A166 (-1.065728, -29.480743) -> (-0.541208, -30.065293) centre (-1.111711, -30.049607) cw
  arc A167 (-1.115535, -29.478901) -> (-1.065728, -29.480743) centre (0, -0.000002) ccw
  arc A168 (-2.19411, -29.418292) -> (-1.115535, -29.478901) centre (0, 0) ccw
  arc A169 (-2.804674, -29.939081) -> (-2.19411, -29.418292) centre (-2.236517, -29.986876) cw
  arc A170 (-4.457708, -33.70651) -> (-2.804674, -29.939081) centre (-9.314173, -29.329275) ccw
  arc A171 (-5.962081, -33.473177) -> (-4.457708, -33.70651) centre (0, 0) ccw
  arc A172 (-6.396257, -29.382012) -> (-5.962081, -33.473177) centre (-0.008364, -30.772717) ccw
  arc A173 (-6.796658, -28.706366) -> (-6.396257, -29.382012) centre (-6.952737, -29.255328) cw
  arc A174 (-6.845149, -28.694842) -> (-6.796658, -28.706366) centre (-0.000001, -0.000002) ccw
  arc A175 (-7.891175, -28.424978) -> (-6.845149, -28.694842) centre (0, 0) ccw
  arc A176 (-8.591608, -28.816645) -> (-7.891175, -28.424978) centre (-8.043692, -28.974364) cw
  arc A177 (-10.947868, -32.189194) -> (-8.591608, -28.816645) centre (-14.857062, -26.948616) ccw
  arc A178 (-12.377814, -31.666855) -> (-10.947868, -32.189194) centre (0, 0) ccw
  arc A179 (-12.005501, -27.569598) -> (-12.377814, -31.666855) centre (-6.011663, -30.179796) ccw
  arc A180 (-12.266396, -26.828819) -> (-12.005501, -27.569598) centre (-12.526574, -27.336783) cw
  arc A181 (-12.311707, -26.808056) -> (-12.266396, -26.828819) centre (-0.000001, -0.000002) ccw
  arc A182 (-13.284986, -26.339308) -> (-12.311707, -26.808056) centre (0, 0) ccw
  arc A183 (-14.048371, -26.586802) -> (-13.284986, -26.339308) centre (-13.541753, -26.848383) cw
  arc A184 (-17.017308, -29.434864) -> (-14.048371, -26.586802) centre (-19.829002, -23.532337) ccw
  arc A185 (-18.317875, -28.643594) -> (-17.017308, -29.434864) centre (0, 0) ccw
  arc A186 (-17.15338, -24.697699) -> (-18.317875, -28.643594) centre (-11.783937, -28.427083) ccw
  arc A187 (-17.264744, -23.920255) -> (-17.15338, -24.697699) centre (-17.619021, -24.367701) cw
  arc A188 (-17.305133, -23.891052) -> (-17.264744, -23.920255) centre (-0.000001, -0.000002) ccw
  arc A189 (-18.168263, -23.241433) -> (-17.305133, -23.891052) centre (0, 0) ccw
  arc A190 (-18.965263, -23.335243) -> (-18.168263, -23.241433) centre (-18.519412, -23.690634) cw
  arc A191 (-22.432782, -25.549369) -> (-18.965263, -23.335243) centre (-24.038924, -19.211724) ccw
  arc A192 (-23.55399, -24.519575) -> (-22.432782, -25.549369) centre (0, 0) ccw
  arc A193 (-21.642065, -20.876681) -> (-23.55399, -24.519575) centre (-17.10336, -25.581932) ccw
  arc A194 (-21.599617, -20.09245) -> (-21.642065, -20.876681) centre (-22.034379, -20.462182) cw
  arc A195 (-21.633533, -20.055928) -> (-21.599617, -20.09245) centre (-0.000002, -0.000002) ccw
  arc A196 (-22.353344, -19.250403) -> (-21.633533, -20.055928) centre (0, 0) ccw
  arc A197 (-23.153331, -19.186923) -> (-22.353344, -19.250403) centre (-22.78538, -19.622467) cw
  arc A198 (-26.986177, -20.682027) -> (-23.153331, -19.186923) centre (-27.325044, -14.152814) ccw
  arc A199 (-27.884939, -19.453283) -> (-26.986177, -20.682027) centre (0, 0) ccw
  arc A200 (-25.299057, -16.253384) -> (-27.884939, -19.453283) centre (-21.765511, -21.753683) ccw
  arc A201 (-25.104429, -15.492503) -> (-25.299057, -16.253384) centre (-25.602968, -15.770313) cw
  arc A202 (-25.130568, -15.450066) -> (-25.104429, -15.492503) centre (-0.000002, -0.000001) ccw
  arc A203 (-25.679398, -14.519591) -> (-25.130568, -15.450066) centre (0, 0) ccw
  arc A204 (-26.451629, -14.301261) -> (-25.679398, -14.519591) centre (-26.175719, -14.80022) cw
  arc A205 (-30.502509, -15.019885) -> (-26.451629, -14.301261) centre (-29.561078, -8.55002) ccw
  arc A206 (-31.144284, -13.639412) -> (-30.502509, -15.019885) centre (0, 0) ccw
  arc A207 (-27.98382, -11.005479) -> (-31.144284, -13.639412) centre (-25.591226, -17.089451) ccw
  arc A208 (-27.644492, -10.297188) -> (-27.98382, -11.005479) centre (-28.18765, -10.472399) cw
  arc A209 (-27.66185, -10.250467) -> (-27.644492, -10.297188) centre (-0.000002, -0.000001) ccw
  arc A210 (-28.018607, -9.2308) -> (-27.66185, -10.250467) centre (0, 0) ccw
  arc A211 (-28.733406, -8.866009) -> (-28.018607, -9.2308) centre (-28.560139, -9.409209) cw
  arc A212 (-32.846646, -8.780538) -> (-28.733406, -8.866009) centre (-30.661097, -2.618654) ccw
  arc A213 (-33.206773, -7.301386) -> (-32.846646, -8.780538) centre (0, 0) ccw
  arc A214 (-29.593181, -5.334639) -> (-33.206773, -7.301386) centre (-28.433485, -11.768482) ccw
  arc A215 (-29.122192, -4.706157) -> (-29.593181, -5.334639) centre (-29.689096, -4.772037) cw
  arc A216 (-29.130102, -4.656948) -> (-29.122192, -4.706157) centre (-0.000002, 0) ccw
  arc A217 (-29.281077, -3.587273) -> (-29.130102, -4.656948) centre (0, 0) ccw
  arc A218 (-29.910974, -3.090042) -> (-29.281077, -3.587273) centre (-29.84701, -3.656607) cw
  arc A219 (-33.928505, -2.20376) -> (-29.910974, -3.090042) centre (-30.582826, 3.413346) ccw
  arc A220 (-33.993144, -0.682771) -> (-33.928505, -2.20376) centre (0, 0) ccw
  arc A221 (-30.065293, 0.541208) -> (-33.993144, -0.682771) centre (-30.18306, -5.995256) ccw
  arc A222 (-29.480743, 1.065728) -> (-30.065293, 0.541208) centre (-30.049607, 1.111711) cw
  arc A223 (-29.478901, 1.115535) -> (-29.480743, 1.065728) centre (-0.000002, 0) ccw
extrude "Extrusion1" add sketch "Sketch1 outline for Extrusion1" along normal blind 15
sketch "Sketch3" plane through (0, 0, 0) normal (0, 0, -1) x (-1, 0, 0)
  circle A0 centre (0, 0) radius 4.5
  dimension "d18" = 9
  constraints: 1 centre point, 1 coincident
  measures "d18" diameter of A0
extrude "Extrusion2" cut sketch "Sketch3" against normal blind 15
body "Solid1"
